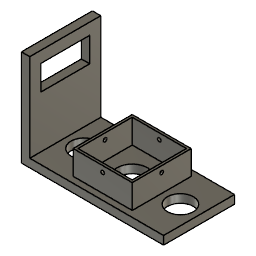
topb (Autodesk Fusion 360 archive; units mm, degrees)
design "topa"
Autodesk Fusion 360 part; units mm, degrees
sketch "Sketch1" plane through (0, 0, 0) normal (0, 0, 1) x (1, 0, 0)
  line L0 (0, 0) -> (22.5, 0)
  line L1 (22.5, 0) -> (22.5, -22.5)
  line L2 (22.5, -22.5) -> (-22.5, -22.5)
  line L3 (-22.5, -22.5) -> (-22.5, 22.5)
  line L4 (-22.5, 22.5) -> (22.5, 22.5)
  line L5 (22.5, 22.5) -> (22.5, 0)
  circle A0 centre (0, 0) radius 12.5
  line L6 (24.5, 0) -> (24.5, -24.5)
  line L7 (24.5, -24.5) -> (-24.5, -24.5)
  line L8 (-24.5, -24.5) -> (-24.5, 24.5)
  line L9 (-24.5, 24.5) -> (24.5, 24.5)
  line L10 (24.5, 24.5) -> (24.5, 0)
  dimension "d1" = 22.5
  dimension "d2" = 22.5
  dimension "d3" = 45
  dimension "d4" = 45
  dimension "d5" = 25
  dimension "d6" = -2
  constraint coincident L0.start A0.centre
  constraint horizontal L0
  constraint perpendicular L0 L1
  constraint perpendicular L1 L2
  constraint perpendicular L2 L3
  constraint perpendicular L3 L4
  constraint perpendicular L0 L5
  measures "d1" distance of L0.start L0.end
  measures "d2" distance of L0.end L1.end
  measures "d3" distance of L1.end L2.end
  measures "d4" distance of L2.end L3.end
  measures "d5" diameter of A0
extrude "Extrude1" add sketch "Sketch1" along normal blind 7 contours L1 L2 L3 L4 L5
extrude "Extrude2" add sketch "Sketch1" along normal blind 27 contours L6 L7 L8 L9 L10
sketch "Sketch2" plane through (0, 0, 0) normal (0, 0, -1) x (1, 0, 0)
  line L0 (-24.5, -24.5) -> (24.5, -24.5)
  line L1 (24.5, -24.5) -> (24.5, 24.5)
  line L2 (24.5, 24.5) -> (-24.5, 24.5)
  line L3 (-24.5, 24.5) -> (-24.5, -24.5)
  circle A0 centre (0, 0) radius 12.5
  line L4 (0, 0) -> (-29.5, 0)
  line L5 (-29.5, 0) -> (-29.5, 29.5)
  line L6 (-29.5, 29.5) -> (29.5, 29.5)
  line L7 (29.5, 29.5) -> (29.5, -29.5)
  line L8 (29.5, -29.5) -> (-29.5, -29.5)
  line L9 (-29.5, -29.5) -> (-29.5, 0)
  line L10 (-29.5, 0) -> (-40, 0)
  line L11 (29.5, 0) -> (40, 0)
  circle A1 centre (-40, 0) radius 10.75
  circle A2 centre (40, 0) radius 10.75
  line L12 (55.5, 29.5) -> (55.5, -29.5)
  line L13 (-55.5, -29.5) -> (-55.5, 0)
  line L14 (-55.5, 0) -> (-55.5, 29.5)
  line L15 (-29.5, -29.5) -> (-55.5, -29.5)
  line L16 (-55.5, 29.5) -> (-29.5, 29.5)
  line L17 (29.5, 29.5) -> (55.5, 29.5)
  line L18 (55.5, -29.5) -> (29.5, -29.5)
  dimension "d11" = 29.5
  dimension "d12" = 29.5
  dimension "d13" = 59
  dimension "d14" = 59
  dimension "d15" = 59
  dimension "d16" = 10.5
  dimension "d17" = 10.5
  dimension "d18" = 21.5
  dimension "d19" = 21.5
  dimension "d20" = -26
  dimension "d21" = -26
  constraint coincident A0.centre L4.start
  constraint perpendicular L3 L4
  constraint perpendicular L4 L5
  constraint perpendicular L5 L6
  constraint perpendicular L2 L7
  constraint perpendicular L3 L8
  constraint perpendicular L5 L10
  constraint midpoint L7 L11.start
  constraint perpendicular L7 L11
  constraint coincident L10.end A1.centre
  constraint coincident L11.end A2.centre
  constraint perpendicular L13 L15
  constraint perpendicular L5 L16
  constraint perpendicular L12 L17
  constraint perpendicular L7 L18
  measures "d11" distance of A0.centre L4.end
  measures "d12" distance of L4.end L5.end
  measures "d13" distance of L5.end L6.end
  measures "d14" distance of L6.end L7.end
  measures "d15" distance of L7.end L8.end
  measures "d16" distance of L4.end L10.end
  measures "d17" distance of L11.start L11.end
  measures "d18" diameter of A1
  measures "d19" diameter of A2
extrude "Extrude3" add sketch "Sketch2" against normal blind 7 contours L5 L6 L7 L8 L9 A1 A2 | L5 L9 A1 L13 L14 L15 L16 | L7 A2 L12 L17 L18
sketch "Sketch3" plane through (0, 0, 0) normal (0, 0, -1) x (1, 0, 0)
  line L0 (55.5, -29.5) -> (55.5, 29.5)
  line L1 (55.5, 29.5) -> (-55.5, 29.5)
  line L2 (-55.5, 29.5) -> (-55.5, -29.5)
  line L3 (-55.5, -29.5) -> (55.5, -29.5)
  circle A0 centre (40, 0) radius 10.75
  circle A1 centre (-40, 0) radius 10.75
  circle A2 centre (0, 0) radius 12.5
  line L4 (-55.5, -29.5) -> (-62.5, -29.5)
  line L5 (-55.5, 29.5) -> (-62.5, 29.5)
  line L6 (-62.5, -29.5) -> (-62.5, 29.5)
  dimension "d24" = 7
  dimension "d25" = 7
  constraint coincident L2.end L3.start
  constraint perpendicular L2 L4
  constraint coincident L1.end L2.start
  constraint perpendicular L5 L6
  measures "d24" distance of L2.end L4.end
  measures "d25" distance of L1.end L5.end
extrude "Extrude4" add sketch "Sketch3" against normal blind 80 contours L2 L4 L5 L6
sketch "Sketch4" plane through (-62.5, 0, 0) normal (-1, 0, 0) x (0, -1, 0)
  line L0 (-29.5, 0) -> (29.5, 0)
  line L1 (29.5, 0) -> (29.5, 80)
  line L2 (29.5, 80) -> (-29.5, 80)
  line L3 (-29.5, 80) -> (-29.5, 0)
  line L4 (29.5, 70.5) -> (-29.5, 70.5)
  line L5 (0, 70.5) -> (20.25, 70.5)
  line L6 (20.25, 70.5) -> (20.25, 50)
  line L7 (20.25, 50) -> (-20.25, 50)
  line L8 (-20.25, 50) -> (-20.25, 70.5)
  line L9 (-20.25, 70.5) -> (20.25, 70.5)
  line L10 (22.25, 72.5) -> (22.25, 48)
  line L11 (22.25, 48) -> (-22.25, 48)
  line L12 (-22.25, 48) -> (-22.25, 72.5)
  line L13 (-22.25, 72.5) -> (22.25, 72.5)
  dimension "d28" = -9.5
  dimension "d29" = 20.25
  dimension "d30" = 20.5
  dimension "d31" = 40.5
  dimension "d32" = -2
  constraint midpoint L4 L5.start
  constraint parallel L4 L5
  constraint perpendicular L5 L6
  constraint perpendicular L6 L7
  constraint coincident L4 L8.end
  constraint perpendicular L4 L8
  constraint coincident L1 L4.start
  constraint coincident L3 L4.end
  measures "d29" distance of L5.start L5.end
  measures "d30" distance of L5.end L6.end
  measures "d31" distance of L6.end L7.end
extrude "Extrude5" cut sketch "Sketch4" against normal blind 7 contours L4 L5 L6 L7 L8 L9
sketch "Sketch5" plane through (24.5, 0, 0) normal (1, 0, 0) x (0, 1, 0)
  line L0 (-24.5, 7) -> (24.5, 7)
  line L1 (24.5, 7) -> (24.5, 27)
  line L2 (24.5, 27) -> (-24.5, 27)
  line L3 (-24.5, 27) -> (-24.5, 7)
  circle A0 centre (0, 22) radius 1.5
  dimension "d35" = 3
  dimension "d36" = 24.5
  dimension "d37" = 15
  measures "d35" diameter of A0
  measures "d36" distance of L3 A0.centre
  measures "d37" distance of L0 A0.centre
sketch "Sketch6" plane through (0, 24.5, 0) normal (0, 1, 0) x (-1, 0, 0)
  line L0 (-24.5, 7) -> (24.5, 7)
  line L1 (24.5, 7) -> (24.5, 27)
  line L2 (24.5, 27) -> (-24.5, 27)
  line L3 (-24.5, 27) -> (-24.5, 7)
  circle A0 centre (0, 22) radius 1.5
  dimension "d38" = 3
  dimension "d39" = 24.5
  dimension "d40" = 15
  measures "d38" diameter of A0
  measures "d39" distance of L3 A0.centre
  measures "d40" distance of L0 A0.centre
extrude "Extrude6" cut sketch "Sketch5" against normal blind 55 contours A0
extrude "Extrude7" cut sketch "Sketch6" against normal blind 55 contours A0
